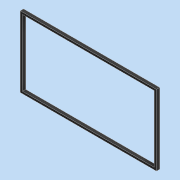
# Autodesk Inventor part: gummi Muttergewinde
Saved by Autodesk Inventor 2021 (Build 250183000, 183)
## iProperties
Created: 2024-03-15
Part Number: gummi Muttergewinde
Material: Generic
Document SubType Name: Modeling
Designer: Nokia
Density: 1 g/cm^3
Appearance: Rubber - Black
Author: Nokia
Autodesk Inventor part; units mm, degrees
ref_plane "YZ Plane" through (0, 0, 0) normal (1, 0, 0) x (0, 1, 0)
ref_plane "XZ Plane" through (0, 0, 0) normal (0, 1, 0) x (-1, 0, 0)
ref_plane "XY Plane" through (0, 0, 0) normal (0, 0, 1) x (1, 0, 0)
sketch "Sketch1" plane through (0, 0, 0) normal (0, 0, 1) x (1, 0, 0)
  line L0 (0, 20) -> (0, 150)
  line L1 (0, 150) -> (-250, 150)
  line L2 (-250, 150) -> (-250, 20)
  line L3 (-250, 20) -> (0, 20)
  line L4 (-4, 24) -> (-246, 24)
  line L5 (-246, 24) -> (-246, 146)
  line L6 (-246, 146) -> (-4, 146)
  line L7 (-4, 146) -> (-4, 24)
  point P0 (0, 0)
  dimension "d2" = 250
  dimension "d3" = 130
  dimension "d4" = 4
  dimension "d5" = 4
  dimension "d6" = 4
  dimension "d7" = 4
  dimension "d10" = 0
  dimension "d11" = 20
  constraints: 16 end point, 4 perpendicular, 2 parallel, 1 horizontal, 1 other
  measures "d2" distance of L0.end L1.end
  measures "d3" distance of L1.end L2.end
  measures "d4" distance between parallel lines of L1 L6
  measures "d5" distance between parallel lines of L0 L7
  measures "d6" distance between parallel lines of L3 L4
  measures "d7" distance between parallel lines of L5 L2
  measures "d10" distance from line of point (0, 0) L0
  measures "d11" distance from line of point (0, 0) L3
extrude "Extrusion1" add sketch "Sketch1" along normal blind 6
body "Solid1"
